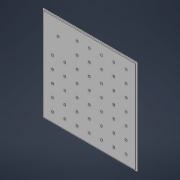
# Autodesk Inventor part: inert låg
Saved by Autodesk Inventor 2022 (Build 260153000, 153)
## iProperties
Created: 2022-10-19
Part Number: inert låg
Material: Generic
Document SubType Name: Modeling
Designer: Jakob Saugbjerg
Density: 1 g/cm^3
Appearance: Default
Author: Jakob Saugbjerg
Autodesk Inventor part; units mm, degrees
ref_plane "YZ Plane" through (0, 0, 0) normal (1, 0, 0) x (0, 1, 0)
ref_plane "XZ Plane" through (0, 0, 0) normal (0, 1, 0) x (-1, 0, 0)
ref_plane "XY Plane" through (0, 0, 0) normal (0, 0, 1) x (1, 0, 0)
sketch "Sketch2" plane through (0, 0, 0) normal (0, 0, 1) x (1, 0, 0)
  line L0 (0, 0) -> (220, 0)
  line L1 (220, 0) -> (220, 220)
  line L2 (220, 220) -> (0, 220)
  line L3 (0, 220) -> (0, 0)
  dimension "d0" = 220
  dimension "d1" = 220
  constraints: 8 end point, 2 parallel, 1 horizontal, 1 perpendicular
  measures "d0" distance of L2.end L1.end
  measures "d1" distance of L1.end L0.end
extrude "Extrusion1" add sketch "Sketch2" along normal blind 3
sketch "Sketch3" plane through (0, 0, 3) normal (0, 0, 1) x (1, 0, 0)
  line L0 (3, 3) -> (217, 3)
  line L1 (217, 3) -> (217, 217)
  line L2 (217, 217) -> (3, 217)
  line L3 (3, 217) -> (3, 3)
  line L4 (3, 3) -> (217, 217) construction
  line L5 (217, 3) -> (3, 217) construction
  line L6 (0, 220) -> (220, 220)
  line L7 (220, 220) -> (220, 0)
  line L8 (220, 0) -> (0, 0)
  line L9 (0, 0) -> (0, 220)
  point P0 (110, 110)
  dimension "d4" = 214
  dimension "d5" = 214
  dimension "d6" = 220
  dimension "d7" = 220
  constraints: 20 end point, 4 parallel, 2 horizontal, 2 midpoint, 2 perpendicular, 1 point on line
  measures "d4" distance of L2.end L1.end
  measures "d5" distance of L1.end L0.end
  measures "d6" distance of L7.end L8.end
  measures "d7" distance of L6.end L7.end
extrude "Extrusion2" cut sketch "Sketch3" against normal blind 1.5
sketch "Sketch4" plane through (0, 0, 0) normal (0, 0, -1) x (-1, 0, 0)
  line L0 (-210, 10) -> (-10, 10)
  line L1 (-10, 10) -> (-10, 210)
  line L2 (-10, 210) -> (-210, 210)
  line L3 (-210, 210) -> (-210, 10)
  line L4 (-210, 10) -> (-10, 210) construction
  line L5 (-10, 10) -> (-210, 210) construction
  line L6 (-210, 10) -> (-181.5, 10)
  line L7 (-181.5, 10) -> (-181.5, 38.5)
  line L8 (-181.5, 38.5) -> (-210, 38.5)
  line L9 (-210, 38.5) -> (-210, 10)
  circle A0 centre (-195.75, 24.25) radius 2.5
  point P0 (0, 0)
  point P1 (-110, 110)
  dimension "d10" = 200
  dimension "d11" = 200
  dimension "d12" = 28.5
  dimension "d13" = 28.5
  dimension "d14" = 5
  constraints: 20 end point, 4 parallel, 2 horizontal, 2 midpoint, 2 perpendicular, 1 centre point, 1 point on line
  measures "d10" distance of L2.end L1.end
  measures "d11" distance of L1.end L0.end
  measures "d12" distance of L8.end L7.end
  measures "d13" distance of L7.end L6.end
  measures "d14" diameter of A0
extrude "Extrusion3" cut sketch "Sketch4" against normal blind 3 contours A0
pattern_linear "Rectangular Pattern1" count 5 spacing 28.5 along (0, 1, 0) count 7 spacing 28.5 along (-1, 0, 0) of "Extrusion3"
sketch "Sketch5" plane through (0, 0, 0) normal (0, 0, -1) x (-1, 0, 0)
  circle A0 centre (-195.75, 138.25) radius 2.5 projected
  line L0 (-195.75, 138.25) -> (-195.75, 166.75)
  circle A1 centre (-195.75, 166.75) radius 2.5
  point P0 (0, 0)
  dimension "d23" = 28.5
  dimension "d24" = 5
  constraints: 2 end point, 1 centre point, 1 coincident, 1 vertical
  measures "d23" distance of L0.start L0.end
  measures "d24" diameter of A1
extrude "Extrusion4" cut sketch "Sketch5" against normal blind 3 contours A1
pattern_linear "Rectangular Pattern2" count 5 spacing 28.5 along (-1, 0, 0) count 2 spacing 28.5 along (0, 1, 0) of "Extrusion4"
sketch "Sketch6" plane through (0, 0, 0) normal (0, 0, -1) x (-1, 0, 0)
  line L0 (-10, 10) -> (-210, 10)
  line L1 (-210, 10) -> (-210, 210)
  line L2 (-210, 210) -> (-10, 210)
  line L3 (-10, 210) -> (-10, 10)
  line L4 (-10, 10) -> (-210, 210) construction
  line L5 (-210, 10) -> (-10, 210) construction
  line L6 (-10, 210) -> (-65, 210)
  line L7 (-65, 210) -> (-65, 155)
  line L8 (-65, 155) -> (-10, 155)
  line L9 (-10, 155) -> (-10, 210)
  circle A0 centre (-37.5, 182.5) radius 2.5
  point P0 (0, 0)
  point P1 (-110, 110)
  dimension "d33" = 200
  dimension "d34" = 200
  dimension "d35" = 55
  dimension "d36" = 55
  dimension "d37" = 5
  constraints: 20 end point, 4 parallel, 2 horizontal, 2 midpoint, 2 perpendicular, 1 centre point, 1 point on line
  measures "d33" distance of L1.end L2.end
  measures "d34" distance of L0.end L1.end
  measures "d35" distance of L8.end L7.end
  measures "d36" distance of L7.end L6.end
  measures "d37" diameter of A0
extrude "Extrusion5" cut sketch "Sketch6" against normal blind 3 contours A0
sketch "Sketch7" plane through (0, 0, 0) normal (0, 0, -1) x (-1, 0, 0)
  point P0 (0, 0)
body "Solid1"
